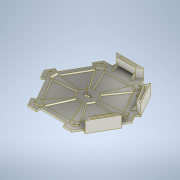
# Autodesk Inventor part: HexagoneBack
Saved by Autodesk Inventor 2020 (Build 240168000, 168)
## iProperties
Created: 2020-04-08
Part Number: HexagoneBack
Material: Silver
Document SubType Name: Modeling
Designer: Samuele
Density: 10.49 g/cm^3
Appearance: Silver
Author: Samuele
## iProperties of the stored document _3DPrint.ipt
Created: 2020-04-27
Part Number: _3DPrint
Material: Generic
Document SubType Name: Modeling
Designer: Samuele
Density: 1 g/cm^3
Appearance: Default
Author: Samuele
Autodesk Inventor part; units mm, degrees
ref_plane "YZ Plane" through (0, 0, 0) normal (1, 0, 0) x (0, 1, 0)
ref_plane "XZ Plane" through (0, 0, 0) normal (0, 1, 0) x (-1, 0, 0)
ref_plane "XY Plane" through (0, 0, 0) normal (0, 0, 1) x (1, 0, 0)
sketch "Sketch6" plane through (0, 0, 0) normal (0, 1, 0) x (-1, 0, 0)
  line L0 (102.5, -48.5) -> (-37.5, -48.5)
  line L1 (32.5, -118.5) -> (32.5, 21.5)
  line L2 (102.5, -48.5) -> (67.5, -109.1218)
  line L3 (67.5, -109.1218) -> (-2.5, -109.1218)
  line L4 (-2.5, -109.1218) -> (-37.5, -48.5)
  line L5 (-37.5, -48.5) -> (-2.5, 12.1218)
  line L6 (-2.5, 12.1218) -> (67.5, 12.1218)
  line L7 (67.5, 12.1218) -> (102.5, -48.5)
  line L8 (32.5, 12.1218) -> (85, -18.1891)
  line L9 (85, -18.1891) -> (85, -78.8109)
  line L10 (85, -78.8109) -> (32.5, -109.1218)
  line L11 (32.5, -109.1218) -> (-20, -78.8109)
  line L12 (-20, -78.8109) -> (-20, -18.1891)
  line L13 (-20, -18.1891) -> (32.5, 12.1218)
  line L14 (32.5, 12.1218) -> (47.5, 12.1218)
  line L15 (47.5, 12.1218) -> (47.5, 5.6218)
  line L16 (47.5, 5.6218) -> (17.5, 5.6218)
  line L17 (17.5, 5.6218) -> (17.5, 12.1218)
  line L18 (47.5, 5.6218) -> (56.6924, 5.6218) construction
  line L19 (17.5, 8.8718) -> (20, 8.8718)
  line L20 (47.5, 8.8718) -> (45, 8.8718)
  line L21 (45, 8.8718) -> (45, 10.1218)
  line L22 (45, 10.1218) -> (20, 10.1218)
  line L23 (20, 10.1218) -> (20, 7.6218)
  line L24 (20, 7.6218) -> (45, 7.6218)
  line L25 (45, 7.6218) -> (45, 10.1218)
  line L26 (67.5, 12.1218) -> (32.5, -48.5)
  line L27 (32.5, -48.5) -> (67.5, -109.1218)
  line L28 (47.5, 5.6218) -> (56.6924, 5.6218)
  line L29 (17.5, 5.6218) -> (11, 5.6218)
  line L30 (17.5, 12.1218) -> (11, 5.6218)
  line L31 (17.5, 12.1218) -> (26.6924, 12.1218) construction
  line L32 (47.5, 12.1218) -> (54, 5.6218)
  line L33 (85, -18.1891) -> (77.5, -5.1987)
  line L34 (77.5, -5.1987) -> (71.8708, -8.4487)
  line L35 (71.8708, -8.4487) -> (86.8708, -34.4295)
  line L36 (86.8708, -34.4295) -> (92.5, -31.1795)
  line L37 (71.8708, -8.4487) -> (67.2746, -0.4879) construction
  line L38 (89.6854, -32.8045) -> (88.4354, -30.6394)
  line L39 (74.6854, -6.8237) -> (75.9354, -8.9888)
  line L40 (75.9354, -8.9888) -> (77.0179, -8.3638)
  line L41 (77.0179, -8.3638) -> (89.5179, -30.0144)
  line L42 (89.5179, -30.0144) -> (87.3529, -31.2644)
  line L43 (87.3529, -31.2644) -> (74.8529, -9.6138)
  line L44 (74.8529, -9.6138) -> (77.0179, -8.3638)
  line L45 (71.8708, -8.4487) -> (67.2746, -0.4879)
  line L46 (86.8708, -34.4295) -> (90.1208, -40.0587)
  line L47 (92.5, -31.1795) -> (90.1208, -40.0587)
  line L48 (92.5, -31.1795) -> (87.9038, -23.2187) construction
  line L49 (77.5, -5.1987) -> (68.6208, -2.8196)
  line L50 (71.8708, -88.5513) -> (67.2746, -96.5121) construction
  line L51 (74.6854, -90.1763) -> (75.9354, -88.0112)
  line L52 (74.8529, -87.3862) -> (77.0179, -88.6362)
  line L53 (77.5, -91.8013) -> (71.8708, -88.5513)
  line L54 (77.5, -91.8013) -> (68.6208, -94.1804)
  line L55 (71.8708, -88.5513) -> (67.2746, -96.5121)
  line L56 (77.0179, -88.6362) -> (89.5179, -66.9856)
  line L57 (87.3529, -65.7356) -> (74.8529, -87.3862)
  line L58 (71.8708, -88.5513) -> (86.8708, -62.5705)
  line L59 (89.5179, -66.9856) -> (87.3529, -65.7356)
  line L60 (89.6854, -64.1955) -> (88.4354, -66.3606)
  line L61 (86.8708, -62.5705) -> (92.5, -65.8205)
  line L62 (86.8708, -62.5705) -> (90.1208, -56.9413)
  line L63 (92.5, -65.8205) -> (90.1208, -56.9413)
  line L64 (94.9944, -48.5) -> (63.7472, -102.6218)
  line L65 (-29.9944, -48.5) -> (1.2528, 5.6218)
  line L66 (1.2528, 5.6218) -> (63.7472, 5.6218)
  line L67 (63.7472, 5.6218) -> (94.9944, -48.5)
  line L68 (32.5, -109.1218) -> (32.5, -115.6218)
  line L69 (32.5, -115.6218) -> (54, -115.6218)
  line L70 (47.5, -115.6218) -> (47.5, -109.1218)
  line L71 (32.5, -115.6218) -> (11, -115.6218)
  line L72 (17.5, -115.6218) -> (17.5, -109.1218)
  line L73 (54, -115.6218) -> (54, -109.1218)
  line L74 (11, -115.6218) -> (11, -109.1218)
  line L75 (90.1208, -40.0587) -> (95.75, -36.8087)
  line L76 (68.6208, -2.8196) -> (74.25, 0.4304)
  line L77 (90.1208, -56.9413) -> (95.75, -60.1913)
  line L78 (68.6208, -94.1804) -> (74.25, -97.4304)
  line L79 (11, 5.6218) -> (11, 12.1218)
  line L80 (54, 5.6218) -> (54, 12.1218)
  line L81 (32.5, -109.1218) -> (32.5, -111.1218)
  line L82 (32.5, -111.1218) -> (45.5, -111.1218)
  line L83 (45.5, -111.1218) -> (45.5, -113.6218)
  line L84 (45.5, -113.6218) -> (19.5, -113.6218)
  line L85 (19.5, -113.6218) -> (19.5, -111.1218)
  line L86 (19.5, -111.1218) -> (32.5, -111.1218)
  line L87 (32.5, -48.5) -> (-2.5, -109.1218)
  line L88 (32.5, -48.5) -> (-2.5, 12.1218)
  line L89 (-20, -78.8109) -> (-25.6292, -82.0609)
  line L90 (-25.6292, -82.0609) -> (-36.3792, -63.4413)
  line L91 (-33.1292, -69.0705) -> (-27.5, -65.8205)
  line L92 (-25.6292, -82.0609) -> (-14.8792, -100.6804)
  line L93 (-18.1292, -95.0513) -> (-12.5, -91.8013)
  line L94 (-36.3792, -63.4413) -> (-30.75, -60.1913)
  line L95 (-14.8792, -100.6804) -> (-9.25, -97.4304)
  line L96 (-20, -78.8109) -> (-21.7321, -79.8109)
  line L97 (-21.7321, -79.8109) -> (-28.2321, -68.5526)
  line L98 (-28.2321, -68.5526) -> (-30.3971, -69.8026)
  line L99 (-30.3971, -69.8026) -> (-17.3971, -92.3192)
  line L100 (-17.3971, -92.3192) -> (-15.2321, -91.0692)
  line L101 (-15.2321, -91.0692) -> (-21.7321, -79.8109)
  line L102 (-20, -18.1891) -> (-25.6292, -14.9391)
  line L103 (-25.6292, -14.9391) -> (-36.3792, -33.5587)
  line L104 (-33.1292, -27.9295) -> (-27.5, -31.1795)
  line L105 (-25.6292, -14.9391) -> (-14.8792, 3.6804)
  line L106 (-18.1292, -1.9487) -> (-12.5, -5.1987)
  line L107 (-15.2321, -5.9308) -> (-21.7321, -17.1891)
  line L108 (-20, -18.1891) -> (-21.7321, -17.1891)
  line L109 (-21.7321, -17.1891) -> (-28.2321, -28.4474)
  line L110 (-14.8792, 3.6804) -> (-9.25, 0.4304)
  line L111 (-36.3792, -33.5587) -> (-30.75, -36.8087)
  line L112 (-17.3971, -4.6808) -> (-15.2321, -5.9308)
  line L113 (-28.2321, -28.4474) -> (-30.3971, -27.1974)
  line L114 (-30.3971, -27.1974) -> (-17.3971, -4.6808)
  line L115 (-29.3146, -27.8224) -> (-30.3146, -29.5545)
  line L116 (-29.3146, -69.1776) -> (-30.3146, -67.4455)
  line L117 (-16.3146, -91.6942) -> (-15.3146, -93.4263)
  line L118 (19.5, -112.3718) -> (17.5, -112.3718)
  line L119 (45.5, -112.3718) -> (47.5, -112.3718)
  line L120 (-15.3146, -3.5737) -> (-16.3146, -5.3058)
  line L121 (19.5, -111.1218) -> (19.5, -109.1218)
  line L122 (45.5, -111.1218) -> (45.5, -109.1218)
  line L123 (-15.2321, -91.0692) -> (-13.5, -90.0692)
  line L124 (-28.2321, -68.5526) -> (-26.5, -67.5526)
  line L125 (-15.2321, -5.9308) -> (-13.5, -6.9308)
  line L126 (-28.2321, -28.4474) -> (-26.5, -29.4474)
  line L127 (63.7472, -102.6218) -> (1.2528, -102.6218)
  line L128 (1.2528, -102.6218) -> (-29.9944, -48.5)
  line L129 (-29.9944, -48.5) -> (1.2528, 5.6218)
  line L130 (1.2528, 5.6218) -> (63.7472, 5.6218)
  line L131 (63.7472, 5.6218) -> (94.9944, -48.5)
  line L132 (94.9944, -48.5) -> (63.7472, -102.6218)
  line L133 (-29.9944, -48.5) -> (-27.9944, -48.5)
  line L134 (-27.9944, -48.5) -> (2.2528, 3.8897)
  line L135 (2.2528, 3.8897) -> (62.7472, 3.8897)
  line L136 (62.7472, 3.8897) -> (92.9944, -48.5)
  line L137 (92.9944, -48.5) -> (62.7472, -100.8897)
  line L138 (62.7472, -100.8897) -> (2.2528, -100.8897)
  line L139 (2.2528, -100.8897) -> (-27.9944, -48.5)
  line L140 (32.5, -48.5) -> (56.7472, -102.6218)
  line L141 (32.5, -48.5) -> (67.2472, -96.5596)
  line L142 (62.7472, -100.8897) -> (60.7472, -97.4256)
  line L143 (60.7472, -97.4256) -> (66.1352, -95.0216)
  line L144 (60.7472, -97.4256) -> (55.9712, -100.8897)
  line L145 (63.7472, -102.6218) -> (62.2472, -100.0237)
  circle A0 centre (62.2472, -100.0237) radius 1.5
  circle A1 centre (32.5, -48.5) radius 10
  circle A2 centre (32.5, -48.5) radius 15
  line L146 (22.5, -48.5) -> (27.5, -39.8397)
  line L147 (27.5, -39.8397) -> (37.5, -39.8397)
  line L148 (37.5, -39.8397) -> (42.5, -48.5)
  line L149 (42.5, -48.5) -> (37.5, -57.1603)
  line L150 (37.5, -57.1603) -> (27.5, -57.1603)
  line L151 (27.5, -57.1603) -> (22.5, -48.5)
  line L152 (17.5, -48.5) -> (25, -35.5096)
  line L153 (25, -35.5096) -> (40, -35.5096)
  line L154 (40, -35.5096) -> (47.5, -48.5)
  line L155 (47.5, -48.5) -> (40, -61.4904)
  line L156 (40, -61.4904) -> (25, -61.4904)
  line L157 (25, -61.4904) -> (17.5, -48.5)
  line L158 (32.5, -48.5) -> (29, -48.5)
  circle A3 centre (29, -48.5) radius 2
  line L159 (29, -46.5) -> (32.1277, -46.5)
  line L160 (29, -50.5) -> (32.1277, -50.5)
  circle A4 centre (35, -48.5) radius 3.5
  line L161 (47.5, -109.1218) -> (17.5, -109.1218)
  line L162 (47.5, -115.6218) -> (53.9, -115.6218)
  line L163 (47.5, -115.6218) -> (47.5, -109.2218)
  line L164 (47.5, -109.2218) -> (53.9, -115.6218)
  line L165 (17.5, -115.6218) -> (17.5, -109.1218)
  line L166 (17.5, -115.6218) -> (11.1, -115.6218)
  line L167 (17.5, -115.6218) -> (17.5, -109.2218)
  line L168 (17.5, -109.2218) -> (11.1, -115.6218)
  line L169 (17.5, -109.2218) -> (47.5, -109.2218)
  line L170 (-12.5866, -91.8513) -> (-14.9292, -100.5938)
  line L171 (-27.5866, -65.8705) -> (-12.5866, -91.8513)
  line L172 (-18.1292, -95.0513) -> (-12.5866, -91.8513)
  line L173 (-33.1292, -69.0705) -> (-27.5866, -65.8705)
  line L174 (-27.5866, -65.8705) -> (-36.3292, -63.5279)
  line L175 (-27.5866, -31.1295) -> (-36.3292, -33.4721)
  line L176 (-12.5866, -5.1487) -> (-27.5866, -31.1295)
  line L177 (-33.1292, -27.9295) -> (-27.5866, -31.1295)
  line L178 (-18.1292, -1.9487) -> (-12.5866, -5.1487)
  line L179 (-12.5866, -5.1487) -> (-14.9292, 3.5938)
  line L180 (88.9944, -48.5) -> (89.6065, -54.3682)
  line L181 (32.5, -48.5) -> (91.4944, -54.5622)
  circle A5 centre (91.9944, -48.5) radius 1.5
  line L182 (88.9944, -48.5) -> (89.6065, -42.6318)
  line L183 (32.5, -48.5) -> (91.4944, -42.4378)
  line L184 (60.7472, 0.4256) -> (66.1352, -1.9784)
  line L185 (32.5, -48.5) -> (67.2472, -0.4404)
  circle A6 centre (62.2472, 3.0237) radius 1.5
  line L186 (60.7472, 0.4256) -> (55.9712, 3.8897)
  line L187 (32.5, -48.5) -> (56.7472, 5.6218)
  line L188 (4.2528, 0.4256) -> (9.0288, 3.8897)
  line L189 (32.5, -48.5) -> (8.2528, 5.6218)
  circle A7 centre (2.7528, 3.0237) radius 1.5
  line L190 (4.2528, 0.4256) -> (-1.1352, -1.9784)
  line L191 (32.5, -48.5) -> (-2.2472, -0.4404)
  line L192 (-23.9944, -48.5) -> (-24.6065, -42.6318)
  line L193 (32.5, -48.5) -> (-26.4944, -42.4378)
  circle A8 centre (-26.9944, -48.5) radius 1.5
  line L194 (-23.9944, -48.5) -> (-24.6065, -54.3682)
  line L195 (32.5, -48.5) -> (-26.4944, -54.5622)
  line L196 (4.2528, -97.4256) -> (-1.1352, -95.0216)
  line L197 (32.5, -48.5) -> (-2.2472, -96.5596)
  circle A9 centre (2.7528, -100.0237) radius 1.5
  line L198 (4.2528, -97.4256) -> (9.0288, -100.8897)
  line L199 (32.5, -48.5) -> (8.2528, -102.6218)
  line L200 (63.422, -91.2689) -> (85, -53.8948)
  line L201 (85, -43.1052) -> (63.422, -5.7311)
  line L202 (54.078, -0.3363) -> (10.922, -0.3363)
  line L203 (1.578, -5.7311) -> (-20, -43.1052)
  line L204 (-20, -53.8948) -> (1.578, -91.2689)
  line L205 (10.922, -96.6637) -> (54.078, -96.6637)
  point P0 (32.5, -48.5)
  point P1 (-13.5, -6.9308)
  point P2 (-26.5, -29.4474)
  point P3 (-13.5, -90.0692)
  point P4 (-26.5, -67.5526)
  point P5 (45.5, -109.1218)
  point P6 (63.6096, -99.3961)
  point P7 (61.0225, -100.8897)
  point P8 (40.8401, -60.0353)
  point P9 (38.3591, -56.6038)
  point P10 (38.06, -56.1902)
  point P11 (36.3799, -57.1603)
  point P12 (63.422, -91.2689)
  point P13 (38.6328, -62.189)
  point P14 (26.3672, -62.189)
  point P15 (23.7114, -60.6557)
  point P16 (17.5786, -50.0333)
  point P17 (17.5786, -46.9667)
  point P18 (23.7114, -36.3443)
  point P19 (26.3672, -34.811)
  point P20 (38.6328, -34.811)
  point P21 (41.2886, -36.3443)
  point P22 (47.4214, -46.9667)
  point P23 (47.4214, -50.0333)
  point P24 (41.2886, -60.6557)
  point P25 (24.1599, -60.0353)
  point P26 (18.3401, -49.9551)
  point P27 (38.3199, -61.4904)
  point P28 (26.6801, -61.4904)
  point P29 (46.6599, -49.9551)
  point P30 (40.8401, -36.9647)
  point P31 (46.6599, -47.0449)
  point P32 (26.6801, -35.5096)
  point P33 (38.3199, -35.5096)
  point P34 (18.3401, -47.0449)
  point P35 (24.1599, -36.9647)
  dimension "d142" = 20
  dimension "d143" = 30
  dimension "d87" = 15
  dimension "d88" = 6.5
  dimension "d91" = 2.5
  dimension "d92" = 2.5
  dimension "d95" = 1.25
  dimension "d96" = 25
  dimension "d97" = 2.5
  dimension "d98" = 25
  dimension "d99" = 135
  dimension "d100" = 0
  dimension "d105" = 30
  dimension "d108" = 6.5
  dimension "d112" = 15
  dimension "d113" = 2
  dimension "d114" = 13
  dimension "d115" = 2.5
  dimension "d116" = 26
  dimension "d118" = 70
  dimension "d119" = 54.1218
  dimension "d120" = 1.25
  dimension "d127" = 2
  dimension "d130" = 7
  dimension "d136" = 4
  dimension "d138" = 3
  dimension "d139" = 3
  dimension "d145" = 3.5
  dimension "d146" = 4
  dimension "d149" = 7
  dimension "d150" = 2.5
  dimension "d152" = 6.5
  dimension "d154" = 6.4
  dimension "d157" = 120
  dimension "d161" = 360
  constraints: 412 end point, 79 symmetric about line, 73 point on line, 17 midpoint, 14 perpendicular, 12 coincident, 9 horizontal, 8 centre point, 2 collinear, 2 equal length, 2 point on circle, 2 tangent, 2 vertical, 1 horizontal alignment, 1 parallel, 191 other
  measures "d87" distance of L8.start L14.end
  measures "d88" distance of L14.end L15.end
  measures "d91" distance of L19.start L19.end
  measures "d92" distance of L20.start L20.end
  measures "d95" distance of L20.end L21.end
  measures "d96" distance of L21.end L22.end
  measures "d97" distance of L22.end L23.end
  measures "d98" distance of L23.end L24.end
  measures "d99" angle of L30 L31
  measures "d100" distance of L17.end L30.start
  measures "d105" distance of L17.end L14.end
  measures "d108" distance of L10.end L68.end
  measures "d112" distance between parallel lines of L68 L70
  measures "d113" distance of L10.end L81.end
  measures "d114" distance of L81.end L82.end
  measures "d115" distance of L82.end L83.end
  measures "d116" distance of L83.end L84.end
  measures "d118" distance of L0.start L2.end
  measures "d119" vertical distance of L66.end L64.start
  measures "d120" vertical distance of L112.start L112.end
  measures "d127" distance of L128.end L133.end
  measures "d130" distance of L140.end L64.end
  measures "d136" distance of L137.end L142.end
  measures "d138" distance of L64.end L145.end
  measures "d139" diameter of A0
  measures "d145" distance of L158.start L158.end
  measures "d146" diameter of A3
  measures "d149" diameter of A4
  measures "d150" distance of point (32.5, -48.5) A4.centre
  measures "d152" distance between parallel lines of L70 L73
  measures "d154" distance of L70.start L163.end
extrude "Plate" add sketch "Sketch6" against normal blind 3 contours L2 L77 L64 L0 | L0 L67 L75 L7 | L64 L181 L137 A5 L0 | L0 A5 L136 L183 L67 | A5 L137 L0 | L0 L136 A5 | L64 L62 L58 L9 L137 L181 | L183 L136 L9 L35 L46 L67 | L137 A5 L0 | L0 A5 L136 | A5 L0 L182 L136 | L137 L180 L0 A5 | L181 L9 L0 L180 | L137 L9 L181 | L183 L9 L136 | L182 L0 L9 L183 | L137 L10 L200 L9 | L9 L58 L10 L137 | L181 A2 L0 L9 | L200 L141 A2 L181 | L136 L8 L35 L9 | L9 L201 L8 L136 | L9 L0 A2 L183 | L183 A2 L185 L201 | L137 L141 L10 | L10 L58 L55 L64 L141 L137 | L181 L155 A2 | A2 L141 L155 L181 | L141 L143 L27 L10 | L10 L27 A2 L141 | L136 L185 L67 L45 L35 L8 | L8 L185 L136 | L183 L154 L185 A2 | A2 L154 L183 | L185 A2 L26 L8 | L8 L26 L184 L185 | L2 L27 L64 L55 L78 | L76 L45 L67 L26 L7 | L141 L64 L27 A0 L137 | L137 A0 L27 L143 | L155 L181 A1 L0 | L0 A1 L183 L154 | A2 L155 L141 | L155 L141 A1 L181 | L27 L144 L140 L10 | L10 L140 A2 L27 | L184 L26 A6 L136 | L136 A6 L26 L67 L185 | L185 L154 A2 | L183 A1 L185 L154 | L26 A2 L187 L8 | L8 L187 L186 L26 | L3 L10 L127 L27 | L26 L66 L28 L80 L6 | A0 L27 L137 | L137 L27 A0 | L27 A0 L138 L144 | L149 L181 A4 L0 | L148 L183 A1 | L0 A4 L183 L148 | A1 L181 L149 | L155 L27 A1 L141 | L156 L140 A1 L27 | A2 L140 L156 | A1 L141 L149 L181 | L140 L138 L10 | L205 L1 A2 L140 | L10 L138 L1 L205 | A6 L26 L136 | L136 L26 A6 | L186 L135 A6 L26 | L154 L185 A1 L26 | L153 L187 A2 | L26 A1 L187 L153 | L183 L148 L185 A1 | L202 L1 L135 L8 | L8 L135 L187 | L187 A2 L1 L202 | L73 L69 L164 L70 L3 | L127 L140 L138 A0 L27 | L26 A6 L135 L187 L66 | L138 A0 L27 | L27 A0 L138 | L140 L127 L10 L138 | A4 L181 L0 | L0 L183 A4 | L183 A4 L185 L148 | L149 L141 A4 L181 | A1 L149 L141 | L150 L140 A4 L27 | L27 A4 L141 L149 | A1 L140 L150 | A2 L1 L156 L140 | L156 L1 A1 L140 | L10 L127 L1 L138 | L205 L199 A2 L1 | L1 L138 L11 L205 | L135 A6 L26 | L26 A6 L135 | L135 L8 L16 L28 L66 L187 | L148 L185 A4 L26 | L147 L187 A1 | L26 A4 L187 L147 | A1 L185 L148 | L187 L153 L1 A2 | L187 A1 L1 L153 | L135 L1 L16 L8 | L202 L13 L135 L1 | L1 A2 L189 L202 | L70 L169 L122 L3 | L195 A4 L0 | L140 A4 L1 | L189 A4 L1 | L187 A4 L26 | L141 A4 L27 | L199 A4 L87 | L191 A4 L88 | L27 A4 L140 | L181 A4 L141 | L185 A4 L183 | L26 A4 L185 | L1 A4 L187 | L88 A4 L189 | L193 A4 L191 | L0 A4 L193 | L197 A4 L195 | L87 A4 L197 | L1 A4 L199 | A1 L1 L150 L140 | L150 L1 A4 L140 | A2 L199 L156 L1 | L156 L199 A1 L1 | L10 L1 L127 | L1 L127 L11 L138 | L199 L198 L87 L11 | L11 L138 L199 | L11 L87 A2 L199 | L187 L147 L1 A1 | L187 A4 L1 L147 | L1 L153 L189 A2 | L1 A1 L189 L153 | L135 L13 L16 L1 | L189 A2 L88 L13 | L189 L135 L13 | L13 L88 L188 L189 | L122 L169 L1 L3 | L164 L69 L70 | L70 L119 L83 L122 L169 | A4 L195 A3 L0 | L0 A3 L193 A4 | L1 L150 L199 L160 A4 | A4 L159 L189 L147 L1 | A4 L199 L160 L87 | L87 L160 L197 A4 | A4 L191 L159 L88 | L88 L159 L189 A4 | L189 L159 A4 | A4 L193 A3 L159 L191 | A4 L197 L160 A3 L195 | A4 L160 L199 | A1 L199 L150 L1 | A2 L156 L199 | L156 L87 A1 L199 | L11 L127 L1 | L1 L169 L121 L3 | L3 L87 L127 L11 | L11 L127 L199 L138 | L87 L196 L197 L11 | L11 L197 A2 L87 | L199 L127 L87 A9 L138 | L138 A9 L87 L198 | L1 L147 L189 A1 | L189 L153 A2 | L189 A1 L88 L153 | L135 L189 L66 L29 L16 L13 | L88 A2 L191 L13 | L13 L191 L190 L88 | L188 L88 A7 L135 | L135 A7 L88 L66 L189 | L122 L82 L1 L169 | L70 L69 L1 L84 L83 L119 | A3 L195 L0 | L0 A3 L193 | L160 L199 L150 L87 | L87 L151 L197 L160 | L159 L191 L146 L88 | L88 L147 L189 L159 | L159 A3 L193 L146 L191 | L193 A3 | A3 L195 | L197 L151 L195 A3 L160 | A1 L150 L199 | L157 L197 A1 L87 | A2 L197 L157 | L1 L86 L121 L169 | L121 L169 L72 L3 | L197 L139 L11 | L204 L195 A2 L197 | L11 L139 L12 L204 | L87 A9 L139 L196 | A9 L87 L138 | L138 L87 A9 | L189 L147 A1 | L152 L191 A2 | L88 A1 L191 L152 | L203 L12 L134 L13 | L13 L134 L191 | L191 A2 L193 L203 | L190 L134 A7 L88 | A7 L88 L135 | L135 L88 A7 | L66 L88 L6 L79 | L83 L84 L1 L82 | L71 L72 L118 L85 L84 L1 | A1 L197 L151 | L146 L191 A1 | L146 L193 A1 L191 | A3 L0 L146 L193 | L195 L151 L0 A3 | L197 A1 L195 L151 | A2 L195 L157 L197 | L157 L195 A1 L197 | L1 L84 L85 L86 | L121 L85 L118 L72 L169 | L72 L168 L71 L74 L3 | L139 L197 L128 L11 | L11 L128 L12 L139 | L139 A9 L87 L128 L197 | L195 L194 L0 L12 | L12 L139 L195 | L12 L0 A2 L195 | L87 L139 A9 | L87 A9 L139 | L87 L4 L11 L128 | L191 L152 L193 A2 | L191 A1 L193 L152 | L134 L12 L65 L13 | L13 L65 L191 L134 | L191 L65 L88 A7 L134 | L193 A2 L0 L12 | L193 L134 L12 | L12 L0 L192 L193 | A7 L134 L88 | L134 A7 L88 | L65 L13 L5 L88 | L71 L168 L72 | L146 A1 L193 | L195 A1 L151 | A2 L157 L195 | L157 L0 A1 L195 | L11 L12 L128 | L12 L128 L195 L139 | L195 L128 L0 A8 L139 | L139 A8 L0 L194 | L193 L152 A2 | L193 A1 L0 L152 | L65 L12 L13 | L134 L193 L65 L12 | L192 L0 A8 L134 | L134 A8 L0 L65 L193 | L5 L106 L179 L105 L110 | L89 L171 L124 L4 | L4 L0 L128 L12 | L4 L123 L171 L89 | A8 L0 L139 | L139 L0 A8 | L95 L92 L170 L93 L4 | L12 L65 L0 L5 | L102 L176 L125 L5 | L5 L126 L176 L102 | A8 L0 L134 | L134 L0 A8 | L5 L125 L176 L106 | L4 L93 L171 L123 | L124 L171 L91 L4 | L171 L123 L101 L89 | L89 L97 L124 L171 | L5 L104 L176 L126 | L176 L126 L109 L102 | L102 L107 L125 L176 | L176 L125 L112 L120 L106 | L106 L105 L179 | L171 L93 L117 L100 L123 | L91 L174 L90 L94 L4 | L124 L98 L116 L91 L171 | L101 L100 L99 L89 | L89 L99 L98 L97 | L170 L92 L93 | L5 L111 L103 L175 L104 | L176 L104 L115 L113 L126 | L109 L113 L114 L102 | L102 L114 L112 L107 | L120 L112 L114 L102 L105 L106 | L91 L90 L174 | L99 L100 L117 L93 L92 L89 | L89 L90 L91 L116 L98 L99 | L175 L103 L104 | L114 L113 L115 L104 L103 L102
extrude "Cazzetti" add sketch "Sketch6" along normal blind 15 contours L164 L69 L70 | L70 L119 L83 L122 L169 | L122 L82 L1 L169 | L70 L69 L1 L84 L83 L119 | L1 L86 L121 L169 | L71 L72 L118 L85 L84 L1 | L121 L85 L118 L72 L169 | L71 L168 L72 | L171 L123 L101 L89 | L89 L97 L124 L171 | L176 L126 L109 L102 | L102 L107 L125 L176 | L176 L125 L112 L120 L106 | L106 L105 L179 | L171 L93 L117 L100 L123 | L124 L98 L116 L91 L171 | L170 L92 L93 | L176 L104 L115 L113 L126 | L120 L112 L114 L102 L105 L106 | L91 L90 L174 | L99 L100 L117 L93 L92 L89 | L89 L90 L91 L116 L98 L99 | L175 L103 L104 | L114 L113 L115 L104 L103 L102
extrude "ScavoStrip" cut sketch "Sketch6" along normal blind 5 contours L122 L169 L1 L3 | L1 L169 L121 L3 | L122 L82 L1 L169 | L1 L86 L121 L169 | L89 L171 L124 L4 | L4 L123 L171 L89 | L102 L176 L125 L5 | L5 L126 L176 L102 | L171 L123 L101 L89 | L89 L97 L124 L171 | L176 L126 L109 L102 | L102 L107 L125 L176
extrude "ScalinoAllineamento" add sketch "Sketch6" along normal blind 2 contours L141 L143 L27 L10 | L141 L64 L27 A0 L137 | L137 A0 L27 L143 | L27 L144 L140 L10 | L27 A0 L138 L144 | L127 L140 L138 A0 L27
extrude "Foro" cut sketch "Sketch6" against normal blind 9.25 contours A0 L27 L137 | L137 L27 A0 | L138 A0 L27 | L27 A0 L138
extrude "ForoMuro" cut sketch "Sketch6" against normal blind 10 contours A4 L181 L0 | L0 L183 A4 | L195 A4 L0 | L140 A4 L1 | L189 A4 L1 | L187 A4 L26 | L141 A4 L27 | L199 A4 L87 | L191 A4 L88 | L27 A4 L140 | L181 A4 L141 | L185 A4 L183 | L26 A4 L185 | L1 A4 L187 | L88 A4 L189 | L193 A4 L191 | L0 A4 L193 | L197 A4 L195 | L87 A4 L197 | L1 A4 L199 | A4 L195 A3 L0 | L0 A3 L193 A4 | A4 L199 L160 L87 | L87 L160 L197 A4 | A4 L191 L159 L88 | L88 L159 L189 A4 | L189 L159 A4 | A4 L193 A3 L159 L191 | A4 L197 L160 A3 L195 | A4 L160 L199 | A3 L195 L0 | L0 A3 L193 | L193 A3 | A3 L195
extrude "Scavi" cut sketch "Sketch6" against normal blind 1.5 contours L200 L141 A2 L181 | L183 A2 L185 L201 | A2 L141 L155 L181 | L183 L154 L185 A2 | L205 L1 A2 L140 | L187 A2 L1 L202 | A2 L1 L156 L140 | L205 L199 A2 L1 | L187 L153 L1 A2 | L1 A2 L189 L202 | A2 L199 L156 L1 | L1 L153 L189 A2 | L204 L195 A2 L197 | L191 A2 L193 L203 | A2 L195 L157 L197 | L191 L152 L193 A2
chamfer "Smussi" distance 2 angle 45 1 edges at (-58.75, 2, -93.9663)
pattern_circular "ScalinoCircolare" count 6 over 360 about axis through (-32.5, 0, -48.5) along (0, 1, 0) of "ScalinoAllineamento", "Foro", "Smussi"
chamfer "Chamfer3" distance 1.5 angle 45 4 edges at (-74.211, -1.5, -72.5819) (-52.1311, -1.5, -75.6521) (-65.83, -1.5, -51.9249) (-43.75, -1.5, -54.9952)
chamfer "Chamfer4" distance 1.5 angle 45 4 edges at (-65.83, -1.5, -45.0751) (-74.211, -1.5, -24.4181) (-43.75, -1.5, -42.0048) (-52.1311, -1.5, -21.3479)
chamfer "Chamfer5" distance 1.5 angle 45 4 edges at (-46.1989, -1.5, -17.9229) (-32.5, -1.5, -35.5096) (-18.8011, -1.5, -17.9229) (-32.5, -1.5, -0.3363)
chamfer "Chamfer6" distance 1.5 angle 45 4 edges at (-21.25, -1.5, -42.0048) (-12.8689, -1.5, -21.3479) (0.83, -1.5, -45.0751) (9.211, -1.5, -24.4181)
chamfer "Chamfer7" distance 1.5 angle 45 4 edges at (0.83, -1.5, -51.9249) (9.211, -1.5, -72.5819) (-12.8689, -1.5, -75.6521) (-21.25, -1.5, -54.9952)
chamfer "Chamfer8" distance 1.5 angle 45 4 edges at (-18.8011, -1.5, -79.0771) (-32.5, -1.5, -61.4904) (-32.5, -1.5, -96.6637) (-46.1989, -1.5, -79.0771)
sketch "Sketch10" plane through (0, 0, 0) normal (0, 1, 0) x (1, 0, 0)
  line L0 (-17.5, 109.2218) -> (-19.5, 109.2218) projected
  line L1 (-17.5, 109.2218) -> (-17.5, 101.2218)
  line L2 (-17.5, 101.2218) -> (-19.5, 101.2218)
  line L3 (-19.5, 101.2218) -> (-19.5, 109.2218)
  line L4 (-45.5, 109.2218) -> (-19.5, 109.2218) projected
  line L5 (-17.5, 109.2218) -> (-19.5, 109.2218)
  line L6 (-54, 115.6218) -> (-11, 115.6218) projected
  line L7 (-32.5, 115.6218) -> (-32.5, 94.111)
  line L8 (-47.5, 109.2218) -> (-45.5, 109.2218)
  line L9 (-47.5, 109.2218) -> (-47.5, 101.2218)
  line L10 (-47.5, 101.2218) -> (-45.5, 101.2218)
  line L11 (-45.5, 101.2218) -> (-45.5, 109.2218)
  line L12 (-47.5, 109.2218) -> (-45.5, 109.2218)
  point P0 (0, 0)
  dimension "d189" = 2
  dimension "d190" = 8
  constraints: 20 end point, 4 symmetric about line, 2 perpendicular, 2 vertical, 1 horizontal, 1 midpoint, 1 point on line
  measures "d189" distance of L1.end L2.end
  measures "d190" distance of L0.start L1.end
extrude "Nervature" add sketch "Sketch10" along normal blind 8
chamfer "SmussoNervature" distance 8 angle 45 2 edges at (-46.5, 8, -101.2218) (-18.5, 8, -101.2218)
pattern_circular "Circular Pattern2" count 3 over 120 about axis through (-32.5, 0, -48.5) along (0, -1, 0) of "Nervature", "SmussoNervature"
body "Solid4"
